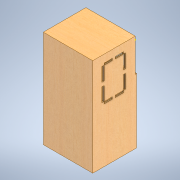
# Autodesk Inventor part: button unit
Saved by Autodesk Inventor 2022.2 (Build 262287000, 287)
## iProperties
Created: 2022-02-27
Part Number: button unit
Material: Pine, Southern
Document SubType Name: Modeling
Designer: PRASHANTH
Density: 0.570257 g/cm^3
Appearance: Yellow Pine - Stained Dark Medium Gloss
Author: PRASHANTH
Autodesk Inventor part; units mm, degrees
ref_plane "YZ Plane" through (0, 0, 0) normal (1, 0, 0) x (0, 1, 0)
ref_plane "XZ Plane" through (0, 0, 0) normal (0, 1, 0) x (-1, 0, 0)
ref_plane "XY Plane" through (0, 0, 0) normal (0, 0, 1) x (1, 0, 0)
sketch "Sketch1" plane through (0, 0, 0) normal (1, 0, 0) x (0, 1, 0)
  line L0 (11.3212, 0) -> (-338.6788, 0)
  line L1 (-338.6788, 0) -> (-338.6788, 150)
  line L2 (-338.6788, 150) -> (11.3212, 150)
  line L3 (11.3212, 150) -> (11.3212, 0)
  point P0 (0, 0)
  dimension "d0" = 350
  dimension "d1" = 150
  constraints: 8 end point, 2 parallel, 1 horizontal, 1 perpendicular
  measures "d0" distance of L1.end L2.end
  measures "d1" distance of L0.end L1.end
extrude "Extrusion1" add sketch "Sketch1" along normal blind 5
sketch "Sketch2" plane through (5, 0, 0) normal (1, 0, 0) x (0, 0, -1)
  line L0 (-150, 11.3212) -> (-150, -338.6788) projected
  line L1 (0, -338.6788) -> (0, 11.3212) projected
  line L2 (-150, 11.3212) -> (0, 11.3212)
  line L3 (0, 11.3212) -> (0, 6.3212)
  line L4 (0, 6.3212) -> (-150, 6.3212)
  line L5 (-150, 6.3212) -> (-150, 11.3212)
  point P0 (0, 0)
  point P1 (0, 11.3212)
  dimension "d4" = 5
  constraints: 8 end point, 2 parallel, 1 horizontal, 1 perpendicular, 1 point on line
  measures "d4" distance of L2.end L3.end
extrude "Extrusion2" add sketch "Sketch2" along normal blind 170
sketch "Sketch3" plane through (0, -338.6788, 150) normal (0, 0, 1) x (1, 0, 0)
  point P0 (0, 338.6788)
sketch "Sketch4" plane through (0, -338.6788, 150) normal (0, 0, 1) x (1, 0, 0)
  line L0 (0, 350) -> (0, 0) projected
  line L1 (0, 350) -> (175.2508, 350)
  line L2 (175.2508, 350) -> (175.2508, 0)
  line L3 (175.2508, 0) -> (0, 0)
  line L4 (0, 0) -> (0, 350)
  point P0 (0, 338.6788)
  constraints: 8 end point, 2 parallel, 1 horizontal, 1 perpendicular
extrude "Extrusion3" add sketch "Sketch4" along normal blind 5
sketch "Sketch5" plane through (175, 0, 0) normal (1, 0, 0) x (0, 0, -1)
  line L0 (0, 11.3212) -> (-155, 11.3212) projected
  line L1 (-155, 11.3212) -> (0, 11.3212)
  line L2 (0, 11.3212) -> (0, -338.6788)
  line L3 (0, -338.6788) -> (-155, -338.6788)
  line L4 (-155, -338.6788) -> (-155, 11.3212)
  point P0 (0, 0)
  constraints: 8 end point, 2 parallel, 1 horizontal, 1 perpendicular
extrude "Extrusion4" add sketch "Sketch5" along normal blind 5
sketch "Sketch6" plane through (0, -338.6788, 0) normal (0, 0, -1) x (-1, 0, 0)
  line L0 (-180, 0) -> (-180, 350) projected
  line L1 (-180, 0) -> (0, 0)
  line L2 (0, 0) -> (0, 230)
  line L3 (0, 230) -> (-180, 230)
  line L4 (-180, 230) -> (-180, 0)
  point P0 (0, 338.6788)
  point P1 (-180, 230)
  dimension "d34" = 230
  constraints: 8 end point, 2 parallel, 1 horizontal, 1 perpendicular
  measures "d34" distance between parallel lines of L1 L3
extrude "Extrusion5" add sketch "Sketch6" along normal blind 5
sketch "Sketch7" plane through (0, -338.6788, 155) normal (0, -1, 0) x (1, 0, 0)
  line L0 (180, -155) -> (180, 0) projected
  line L1 (0, -160) -> (180, -160) projected
  line L2 (180, 0) -> (0, 0)
  line L3 (0, 0) -> (0, -160)
  line L4 (0, -160) -> (180, -160)
  line L5 (180, -160) -> (180, 0)
  point P0 (0, -155)
  constraints: 8 end point, 2 parallel, 1 horizontal, 1 perpendicular
extrude "Extrusion6" add sketch "Sketch7" along normal blind 5
sketch "Sketch8" plane through (180, 0, 0) normal (1, 0, 0) x (0, 0, -1)
  point P0 (0, 0)
sketch "Sketch9" plane through (180, 0, 0) normal (1, 0, 0) x (0, 0, -1)
  line L0 (-113.8942, -23.5999) -> (-43.3942, -23.5999)
  line L1 (-43.3942, -23.5999) -> (-43.3942, -137.9783)
  line L2 (-43.3942, -137.9783) -> (-113.8942, -137.9783)
  line L3 (-113.8942, -137.9783) -> (-113.8942, -23.5999)
  line L4 (-43.3942, -73.5999) -> (-43.3942, -23.5999)
  line L5 (-43.3942, -137.9783) -> (-35.8942, -137.9783)
  line L6 (-35.8942, -137.9783) -> (-35.8942, -87.9783)
  line L7 (-35.8942, -87.9783) -> (-43.3942, -87.9783)
  line L8 (-43.3942, -87.9783) -> (-43.3942, -137.9783)
  line L9 (-43.3942, -65.8129) -> (-43.3942, -23.5999)
  line L10 (-113.8942, -23.5999) -> (-121.3942, -23.5999)
  line L11 (-121.3942, -23.5999) -> (-121.3942, -73.5999)
  line L12 (-121.3942, -73.5999) -> (-113.8942, -73.5999)
  line L13 (-113.8942, -73.5999) -> (-113.8942, -23.5999)
  line L14 (-113.8942, -137.9783) -> (-121.3942, -137.9783)
  line L15 (-121.3942, -137.9783) -> (-121.3942, -87.9783)
  line L16 (-121.3942, -87.9783) -> (-113.8942, -87.9783)
  line L17 (-113.8942, -87.9783) -> (-113.8942, -137.9783)
  line L18 (-113.8942, -137.9783) -> (-83.8942, -137.9783)
  line L19 (-83.8942, -137.9783) -> (-83.8942, -145.4783)
  line L20 (-83.8942, -145.4783) -> (-113.8942, -145.4783)
  line L21 (-113.8942, -145.4783) -> (-113.8942, -137.9783)
  line L22 (-43.3942, -137.9783) -> (-73.3942, -137.9783)
  line L23 (-73.3942, -137.9783) -> (-73.3942, -145.4783)
  line L24 (-73.3942, -145.4783) -> (-43.3942, -145.4783)
  line L25 (-43.3942, -145.4783) -> (-43.3942, -137.9783)
  line L26 (-43.3942, -23.5999) -> (-35.8942, -23.5999)
  line L27 (-35.8942, -23.5999) -> (-35.8942, -73.5999)
  line L28 (-35.8942, -73.5999) -> (-43.3942, -73.5999)
  line L29 (-43.3942, -73.5999) -> (-43.3942, -23.5999)
  line L30 (-113.8942, -23.5999) -> (-83.8942, -23.5999)
  line L31 (-83.8942, -23.5999) -> (-83.8942, -16.6897)
  line L32 (-83.8942, -16.6897) -> (-113.8942, -16.6897)
  line L33 (-113.8942, -16.6897) -> (-113.8942, -23.5999)
  line L34 (-73.3942, -16.0999) -> (-43.3942, -16.0999)
  line L35 (-43.3942, -16.0999) -> (-43.3942, -23.5999)
  line L36 (-43.3942, -23.5999) -> (-73.3942, -23.5999)
  line L37 (-73.3942, -23.5999) -> (-73.3942, -16.0999)
  point P0 (0, 0)
  dimension "d18" = 7.5
  dimension "d19" = 7.5
  dimension "d20" = 30
  dimension "d21" = 30
  dimension "d22" = 7.5
  dimension "d23" = 50
  dimension "d24" = 50
  dimension "d25" = 50
  dimension "d26" = 50
  dimension "d27" = 7.5
  dimension "d28" = 7.5
  dimension "d29" = 30
  dimension "d30" = 30
  dimension "d31" = 7.5
  constraints: 76 end point, 18 parallel, 9 horizontal, 9 perpendicular
  measures "d18" distance of L12.end L11.end
  measures "d19" distance of L15.end L16.end
  measures "d20" distance of L19.end L20.end
  measures "d21" distance of L24.end L23.end
  measures "d22" distance of L27.end L28.end
  measures "d23" distance of L26.end L27.end
  measures "d24" distance of L5.end L6.end
  measures "d25" distance of L14.end L15.end
  measures "d26" distance of L10.end L11.end
  measures "d27" distance of L22.end L23.end
  measures "d28" distance of L18.end L19.end
  measures "d29" distance of L32.end L31.end
  measures "d30" distance of L34.start L34.end
  measures "d31" distance of L36.end L34.start
extrude "Extrusion7" cut sketch "Sketch9" against normal blind 5 contours L33 L32 L31 L0 | L3 L12 L11 L10 | L37 L34 L35 L0 | L3 L14 L15 L16 | L26 L27 L28 L1 | L2 L19 L20 L21 | L2 L25 L24 L23 | L7 L6 L5 L1
sketch "Sketch10" plane through (180, 0, 0) normal (1, 0, 0) x (0, 0, -1)
  point P0 (0, 0)
body "Solid1"
